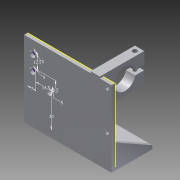
# Autodesk Inventor part: galvo holder
Saved by Autodesk Inventor 2014 (Build 180170000, 170)
## iProperties
Created: 2014-06-21
Part Number: galvo holder
Material: ABS Plastic
Document SubType Name: Modeling
Designer: cruiser
Density: 1.06 g/cm^3
Appearance: Smooth - White
Author: cruiser
Autodesk Inventor part; units mm, degrees
ref_plane "YZ Plane" through (0, 0, 0) normal (1, 0, 0) x (0, 1, 0)
ref_plane "XZ Plane" through (0, 0, 0) normal (0, 1, 0) x (-1, 0, 0)
ref_plane "XY Plane" through (0, 0, 0) normal (0, 0, 1) x (1, 0, 0)
sketch "Sketch1" plane through (0, 0, 0) normal (0, 1, 0) x (-1, 0, 0)
  line L0 (37.5, -31) -> (-37.5, -31)
  line L1 (-37.5, -31) -> (-37.5, 31)
  line L2 (-37.5, 31) -> (37.5, 31)
  line L3 (37.5, 31) -> (37.5, -31)
  line L4 (37.5, -31) -> (-37.5, 31) construction
  line L5 (-37.5, -31) -> (37.5, 31) construction
  point P0 (0, 0)
  dimension "d0" = 75
  dimension "d1" = 62
  constraints: 12 end point, 2 midpoint, 2 parallel, 1 horizontal, 1 perpendicular
  measures "d0" distance of L1.end L2.end
  measures "d1" distance of L0.end L1.end
extrude "Extrusion1" add sketch "Sketch1" along normal blind 3
sketch "Sketch2" plane through (0, 3, 0) normal (0, 1, 0) x (1, 0, 0)
  line L0 (37.5, 31) -> (-37.5, 31) projected
  line L1 (-37.5, 31) -> (-37.5, -31) projected
  circle A0 centre (-30.5, -7.5) radius 2.5
  circle A1 centre (-30.5, -20) radius 2.5
  circle A2 centre (-16, 1) radius 2.5
  line L2 (-37.5, -31) -> (37.5, -31) projected
  line L3 (37.5, -31) -> (37.5, 31) projected
  line L4 (-30.5, -7.5) -> (-30.5, -31)
  point P0 (0, 0)
  dimension "d4" = 5
  dimension "d5" = 5
  dimension "d6" = 12.5
  dimension "d7" = 7
  dimension "d8" = 5
  dimension "d9" = 8.5
  dimension "d10" = 14.5
  dimension "d11" = 30
  constraints: 3 centre point, 2 end point, 2 point on line, 1 parallel
  measures "d4" diameter of A0
  measures "d5" diameter of A1
  measures "d6" distance of L4.start A1.centre
  measures "d7" distance from line of L4.start L1
  measures "d8" diameter of A2
  measures "d9" vertical distance of L4.start A2.centre
  measures "d10" horizontal distance of L4.start A2.centre
  measures "d11" distance from line of L0 A2.centre
extrude "Extrusion2" cut sketch "Sketch2" against normal through all contours A0 | A1 L4 | L4 A1 | A2
sketch "Sketch3" plane through (0, 3, 0) normal (0, 1, 0) x (1, 0, 0)
  line L0 (-37.5, 31) -> (-37.5, -31) projected
  line L1 (37.5, -31) -> (37.5, 31) projected
  line L2 (-37.5, -20) -> (37.5, -20)
  line L3 (19.5, -32.5) -> (27.5, -32.5)
  line L4 (27.5, -32.5) -> (27.5, -7.5)
  line L5 (27.5, -7.5) -> (19.5, -7.5)
  line L6 (19.5, -7.5) -> (19.5, -32.5)
  line L7 (19.5, -32.5) -> (27.5, -7.5) construction
  line L8 (27.5, -32.5) -> (19.5, -7.5) construction
  circle A0 centre (-30.5, -20) radius 2.5 projected
  point P0 (0, 0)
  point P1 (23.5, -20)
  dimension "d16" = 8
  dimension "d21" = 25
  dimension "d22" = 0
  dimension "d74" = 50
  constraints: 14 end point, 3 point on line, 2 midpoint, 2 parallel, 2 perpendicular, 1 horizontal
  measures "d16" distance of L5.end L4.end
  measures "d21" distance between parallel lines of L3 L5
  measures "d22" distance from line of L2 A0.centre
  measures "d74" distance from line of L6 A0.centre
extrude "Extrusion3" add sketch "Sketch3" along normal blind 35 contours L6 L5 L4 L2 | L2 L4 L3 L6
sketch "Sketch4" plane through (27.5, 3, 32.5) normal (1, 0, 0) x (0, 0, -1)
  line L0 (25, 0) -> (1.5, 0) projected
  circle A0 centre (12.5, 18.5) radius 9
  line L1 (0, 35) -> (25, 35) projected
  line L2 (10.6712, 35) -> (14.3288, 35)
  line L3 (14.3288, 35) -> (14.3288, 27.3122)
  line L4 (14.3288, 27.3122) -> (10.6712, 27.3122)
  line L5 (10.6712, 27.3122) -> (10.6712, 35)
  line L6 (12.5, 35) -> (12.5, 0)
  line L7 (16.7228, 27.2139) -> (8.2773, 27.2139)
  line L8 (8.2773, 27.2139) -> (8.2773, 30.5)
  line L9 (8.2773, 30.5) -> (16.7228, 30.5)
  line L10 (16.7228, 30.5) -> (16.7228, 27.2139)
  line L11 (16.7228, 27.2139) -> (8.2773, 30.5) construction
  line L12 (8.2773, 27.2139) -> (16.7228, 30.5) construction
  point P0 (0, 0)
  point P1 (32.5, -3)
  point P2 (12.5, 28.8569)
  dimension "d86" = 18
  dimension "d87" = 18.5
  dimension "d88" = 3.6576
  dimension "d89" = 8.4455
  dimension "d90" = 3.2861
  dimension "d91" = 4.5
  constraints: 22 end point, 4 parallel, 3 midpoint, 3 point on line, 2 horizontal, 2 perpendicular, 2 point on circle, 1 centre point, 1 other
  measures "d86" diameter of A0
  measures "d87" distance from line of A0.centre L0
  measures "d88" distance between parallel lines of L3 L5
  measures "d89" distance of L8.end L9.end
  measures "d90" distance of L9.end L7.start
  measures "d91" distance between parallel lines of L1 L9
extrude "Extrusion4" cut sketch "Sketch4" against normal up to surface (8 mm away) contours A0 L6 L7 | L7 L6 L4 A0 | A0 L7 L6 | L4 L6 A0 | A0 L6 L9 L3 | L7 A0 L4 L6 | L6 L4 A0 | A0 L5 L9 L6 | L9 L6 L1 L3 | L9 L5 L1 L6
sketch "Sketch10" plane through (19.5, 3, 32.5) normal (0, 0, 1) x (1, 0, 0)
  circle A0 centre (4, 31) radius 1.5
  point P0 (6, -5)
  dimension "d49" = 3
  constraints: 1 centre point
  measures "d49" diameter of A0
sketch "Sketch9" plane through (19.5, 3, 32.5) normal (0, 0, 1) x (1, 0, 0)
  circle A0 centre (4, 31) radius 2
  point P0 (6, -5)
  dimension "d48" = 4
  constraints: 1 centre point
  measures "d48" diameter of A0
extrude "Extrusion9" cut sketch "Sketch10" against normal through all
extrude "Extrusion10" cut sketch "Sketch9" against normal up to surface (14.3288 mm away)
sketch "Sketch13" plane through (37.5, 0, -31) normal (0, 0, -1) x (-1, 0, 0)
  line L0 (75, 0) -> (75, 3) projected
  line L1 (0, 0) -> (75, 0)
  line L2 (75, 0) -> (75, 35)
  line L3 (75, 35) -> (0, 35)
  line L4 (0, 35) -> (0, 0)
  point P0 (37.5, 0)
  dimension "d71" = 35
  constraints: 8 end point, 2 parallel, 1 collinear, 1 horizontal, 1 perpendicular
  measures "d71" distance of L1.end L2.end
extrude "Extrusion13" add sketch "Sketch13" along normal blind 3
sketch "Sketch14" plane through (0, 0, 0) normal (0, -1, 0) x (1, 0, 0)
  circle A0 centre (21, 27) radius 1.65
  circle A1 centre (33.5, 27) radius 1.65
  line L0 (33.5, 27) -> (21, 27)
  line L1 (21, 27) -> (21, -6)
  line L2 (21, -6) -> (33.5, -6)
  line L3 (33.5, -6) -> (33.5, 27)
  circle A2 centre (21, -6) radius 1.65
  circle A3 centre (33.5, -6) radius 1.65
  line L4 (37.5, -34) -> (37.5, 31) projected
  point P0 (0, 0)
  point P1 (37.5, -31)
  dimension "d75" = 12.5
  dimension "d76" = 3.3
  dimension "d77" = 3.3
  dimension "d78" = 3.3
  dimension "d79" = 3.3
  dimension "d81" = 33
  dimension "d82" = 25
  dimension "d93" = 4
  constraints: 8 end point, 4 centre point, 3 coincident, 2 parallel, 1 horizontal, 1 perpendicular
  measures "d75" distance of L0.start L0.end
  measures "d76" diameter of A3
  measures "d77" diameter of A1
  measures "d78" diameter of A0
  measures "d79" diameter of A2
  measures "d81" distance of L2.end L0.start
  measures "d82" distance from line of L2 point (37.5, -31)
  measures "d93" distance between parallel lines of L4 L3
extrude "Extrusion14" cut sketch "Sketch14" against normal up to next contours L0 L3 A1 | A1 L3 L0 | A3 L2 L3 | L3 L2 A3
sketch "Sketch15" plane through (37.5, 0, 31) normal (1, 0, 0) x (0, 0, -1)
  line L0 (62, 35) -> (62, 3) projected
  line L1 (0, 3) -> (62, 3) projected
  line L2 (62, 35) -> (44, 3)
  point P0 (31, 0)
  dimension "d94" = 18
  constraints: 2 end point, 1 point on line
  measures "d94" distance of L0.end L2.end
extrude "Extrusion15" add sketch "Sketch15" against normal blind 3
sketch "Sketch16" plane through (-37.5, 0, 31) normal (-1, 0, 0) x (0, 0, 1)
  line L0 (-62, 3) -> (0, 3) projected
  line L1 (-62, 3) -> (-62, 35) projected
  line L2 (-62, 35) -> (-44, 3)
  point P0 (-31, 0)
  dimension "d97" = 18
  constraints: 2 end point, 1 point on line
  measures "d97" distance of L0.start L2.end
extrude "Extrusion16" add sketch "Sketch16" against normal blind 3
sketch "Sketch17" plane through (0, 3, 0) normal (0, -1, 0) x (1, 0, 0)
  line L0 (19.5, 31) -> (27.5, 31) projected
  line L1 (27.5, 32.5) -> (27.5, 31) projected
  line L2 (19.5, 32.5) -> (27.5, 32.5) projected
  line L3 (19.5, 31) -> (19.5, 32.5) projected
  point P0 (0, 0)
extrude "Extrusion17" add sketch "Sketch17" along normal up to surface (3 mm away)
equation "\"d88\" = tslot_screw_width"
equation "\"d89\" = tslot_nut_width"
equation "\"d90\" = tslot_nut_thickness"
equation "\"Acrylic_thickness\" = 3.175"
equation "\"Wood_thickness\" = 5"
equation "\"Acrylic_kerf\" = 0"
equation "\"Wood_kerf\" = 0"
equation "\"resevoir_thickness\" = 12.7"
equation "\"acrylic_height\" = 304.8"
equation "\"acrylic_stopper\" = 125"
equation "\"arm_width\" = 25.4"
equation "\"arm_thickness\" = 1.5875"
equation "\"arm_length\" = 224.5"
equation "\"ball_joint_from_arm\" = 14.5"
equation "\"z_railA_from_screw\" = 35"
equation "\"z_railB_from_screw\" = 35"
equation "\"z_rail_D\" = 8"
equation "\"z_rail_support_hole\" = 5"
equation "\"z_screw_D\" = 8"
equation "\"lmk8uu_hole_space\" = 17"
equation "\"lmk8uu_hole_D\" = 3.3"
equation "\"lmk8uu_OD\" = 15"
equation "\"camera_arm_screw\" = 6.35"
equation "\"carrier_thickness\" = 5"
equation "\"turntable_ID\" = 145"
equation "\"turntable_outside_hole_radius\" = 92.72"
equation "\"turntable_inside_hole_radius\" = 79.16"
equation "\"turntable_hole_D\" = 5.6"
equation "\"oring_ID\" = 19.05"
equation "\"oring_OD\" = 23.8125"
equation "\"drive_set_screw\" = 2.5"
equation "\"drive_set_nut\" = 5"
equation "\"nema17_hole_D\" = 3.3"
equation "\"nema17_hole_space\" = 31"
equation "\"box_lid_from_back\" = 147.5"
equation "\"box_lid_slot_length\" = 0"
equation "\"mirror_thickness\" = 8"
equation "\"laser_angle\" = 25deg"
equation "\"laser_distance\" = 155.47675"
equation "\"m8_rail_height\" = 304.8"
equation "\"print_bed_drill\" = 7.9375"
equation "\"front_frame_inset\" = 28.04"
equation "\"petri_OD\" = 152.4"
equation "\"tslot_screw_length\" = 12.7"
equation "\"tslot_screw_width\" = 3.6576"
equation "\"tslot_nut_width\" = 8.4455"
equation "\"tslot_nut_thickness\" = 3.28612"
equation "\"center_frame_inset\" = 186.36"
equation "\"printer_z\" = 289"
equation "\"frame_tilt\" = 1deg"
equation "\"z_min_from_center\" = 72.6"
equation "\"crane_z\" = 25"
equation "\"tape_thickness\" = 2"
equation "\"tape_keep_out\" = 2"
equation "\"brass_keep_out\" = 8"
equation "\"crane_x\" = 245.2"
equation "\"brass_insert_drill\" = 4"
equation "\"bed_clamp_border\" = 15"
equation "\"tray_boarder\" = 15"
equation "\"motor_spacing\" = 296"
equation "\"threaded_rod_z\" = 203.2"
equation "\"linear_bearing_z\" = 304.8"
equation "\"clear_acrylic\" = 2"
equation "\"thin_acrylic\" = 3"
equation "\"carrier_z2\" = 283.6"
equation "\"carrier_z\" = 258.6"
equation "\"thick_acrylic\" = 5.6"
equation "\"linear_bearing_spacing\" = 216"
equation "\"laser_body_diameter\" = 12"
equation "\"stepper_body_diameter\" = 28"
equation "\"stepper_shaft_diameter\" = 5"
equation "\"m3_diameter\" = 3.15"
equation "\"stepper_screw_space\" = 35"
equation "\"m5_diameter\" = 5.25"
equation "\"subframe_y_offset\" = 27.5"
equation "\"laser_y_offset\" = 18.5"
equation "\"laser_diameter\" = 12"
equation "\"laser_y\" = 35"
equation "\"laser_z\" = 18"
body "Solid1"
